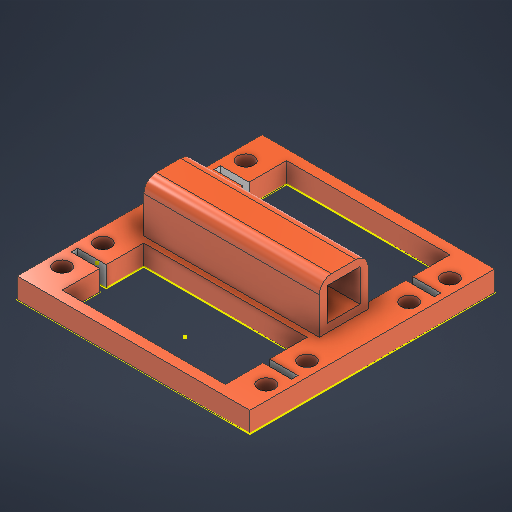
# Autodesk Inventor part: base
Saved by Autodesk Inventor 2027.1 (Build 311270010, 270A)
## iProperties
Created: 2026-08-01
Part Number: base
Material: Ogólny
Document SubType Name: Modeling
Designer: User
Density: 1 g/cm^3
Appearance: Domyślna
Author: User
Autodesk Inventor part; units mm, degrees
ref_plane "YZ Plane" through (0, 0, 0) normal (1, 0, 0) x (0, 1, 0)
ref_plane "XZ Plane" through (0, 0, 0) normal (0, 1, 0) x (-1, 0, 0)
ref_plane "XY Plane" through (0, 0, 0) normal (0, 0, 1) x (1, 0, 0)
sketch "Szkic1" plane through (0, 0, 0) normal (0, 1, 0) x (-1, 0, 0)
  line L0 (0, 0) -> (0, -35)
  circle A0 centre (0, 0) radius 2
  circle A1 centre (0, -35) radius 2
  line L1 (0, 0) -> (0, -35) construction
  line L2 (-25, 0) -> (-25, -35)
  line L3 (25, -35) -> (25, 0)
  arc A2 (25, 0) -> (-25, 0) centre (0, 0) ccw
  arc A3 (-25, -35) -> (25, -35) centre (0, -35) ccw
  line L4 (-20, -45) -> (20, -45)
  line L5 (20, -45) -> (20, -25)
  line L6 (20, -25) -> (-20, -25)
  line L7 (-20, -25) -> (-20, -45)
  line L8 (-20, -45) -> (20, -25) construction
  line L9 (20, -45) -> (-20, -25) construction
  line L10 (0, -17.5) -> (-25, -17.5) construction
  line L11 (0, -35) -> (0, 0)
  circle A4 centre (0, 0) radius 2
  line L12 (0, -35) -> (0, 0) construction
  line L13 (-20, 10) -> (20, 10)
  line L14 (20, 10) -> (20, -10)
  line L15 (20, -10) -> (-20, -10)
  line L16 (-20, 10) -> (20, -10) construction
  line L17 (20, 10) -> (-20, -10) construction
  line L18 (-20, -10) -> (-20, 10)
  line L19 (0, -17.5) -> (-400, -17.5) construction
  line L20 (0, -17.5) -> (400, -17.5) construction
  line L21 (21.5, 12.5) -> (-21.5, 12.5)
  line L22 (-21.5, 12.5) -> (-21.5, -47.5)
  line L23 (-21.5, -47.5) -> (21.5, -47.5)
  line L24 (21.5, -47.5) -> (21.5, 12.5)
  line L25 (21.5, 12.5) -> (-21.5, -47.5) construction
  line L26 (-21.5, 12.5) -> (21.5, -47.5) construction
  line L27 (21.5, -47.5) -> (28.5, -47.5)
  line L28 (28.5, -47.5) -> (28.5, 12.5)
  line L29 (28.5, 12.5) -> (21.5, 12.5)
  line L30 (21.5, 12.5) -> (21.5, -47.5)
  line L31 (20, 10) -> (20, -10)
  line L32 (20, 0) -> (20, -10)
  circle A5 centre (25, -5) radius 2
  line L33 (20, 0) -> (28.5, 0) construction
  circle A6 centre (25, 5) radius 2
  circle A7 centre (-25, -5) radius 2
  circle A8 centre (-25, 5) radius 2
  line L34 (-21.5, -47.5) -> (-21.5, 12.5)
  line L35 (-21.5, -47.5) -> (-28.5, -47.5)
  line L36 (-28.5, -47.5) -> (-28.5, 12.5)
  line L37 (-28.5, 12.5) -> (-21.5, 12.5)
  circle A9 centre (25, -30) radius 2
  circle A10 centre (25, -40) radius 2
  circle A11 centre (-25, -30) radius 2
  circle A12 centre (-25, -40) radius 2
  point P0 (20, -5)
  dimension "d0" = 35
  dimension "d1" = 4
  dimension "d2" = 4
  dimension "d3" = 50
  dimension "d6" = 40
  dimension "d7" = 20
  dimension "d8" = 400
  dimension "d9" = 180
  dimension "d10" = 43
  dimension "d11" = 60
  dimension "d21" = 7
  dimension "d22" = 60
  dimension "d24" = 4
  dimension "d25" = 5
  dimension "d26" = 5
  constraints: 80 end point, 19 symmetric about line, 13 centre point, 8 midpoint, 7 parallel, 5 collinear, 4 coincident, 4 horizontal, 4 perpendicular, 4 point on circle, 4 tangent, 2 vertical, 1 point on line, 8 other
  measures "d0" distance of L0.start L0.end
  measures "d1" diameter of A0
  measures "d2" diameter of A1
  measures "d3" diameter of A3
  measures "d6" distance of L6.end L5.end
  measures "d7" distance of L5.end L4.end
  measures "d8" distance of L10.start L19.end
  measures "d9" angle of L20 L19
  measures "d10" distance of L23.end L22.end
  measures "d11" distance of L22.end L21.end
  measures "d21" distance of L29.end L28.end
  measures "d22" distance of L28.end L27.end
  measures "d24" diameter of A5
  measures "d25" distance from line of L15 A5.centre
  measures "d26" distance of point (20, -5) A5.centre
extrude "Wyciągnięcie proste1" add sketch "Szkic1" against normal blind 5 contours L21 L24 L23 L22
sketch "Szkic2" plane through (-21.5, 0, -47.5) normal (-1, 0, 0) x (0, 0, 1)
  line L0 (22.5, 0) -> (22.5, -5) projected
  line L1 (37.5, 0) -> (37.5, -5) projected
  line L2 (22.5, 0) -> (37.5, 0)
  line L3 (30, 0) -> (30, 6)
  line L4 (36, 12) -> (24, 12)
  line L5 (24, 12) -> (24, 0)
  line L6 (24, 0) -> (36, 0)
  line L7 (36, 0) -> (36, 12)
  line L8 (36, 12) -> (24, 0) construction
  line L9 (24, 12) -> (36, 0) construction
  line L10 (34, 10) -> (26, 10)
  line L11 (26, 10) -> (26, 2)
  line L12 (26, 2) -> (34, 2)
  line L13 (34, 2) -> (34, 10)
  line L14 (34, 10) -> (26, 2) construction
  line L15 (26, 10) -> (34, 2) construction
  point P0 (47.5, 0)
  point P1 (36, 0)
  point P2 (24, 0)
  dimension "d12" = 6
  dimension "d13" = 12
  dimension "d14" = 12
  dimension "d15" = 8
  dimension "d16" = 8
  constraints: 28 end point, 5 midpoint, 4 parallel, 3 horizontal, 2 perpendicular, 1 vertical
  measures "d12" distance of L3.start L3.end
  measures "d13" distance of L6.end L5.end
  measures "d14" distance of L5.end L4.end
  measures "d15" distance of L12.end L11.end
  measures "d16" distance of L11.end L10.end
extrude "Wyciągnięcie proste2" add sketch "Szkic2" against normal up to surface (43 mm away)
fillet "Zaokrąglenie2" radius 3 2 edges at (0, 12, -11.5) (0, 12, -23.5)
extrude "Wyciągnięcie proste3" add sketch "Szkic1" against normal blind 5 contours A2 A8 L37 L22 L35 A3 A12 L2 A11 A7 | L2 A7 A11 A3 A12 L35 L36 L37 A2 A8 | L29 L28 L27 A3 A10 L3 A9 A5 A2 A6 | A2 A6 L3 A5 A9 A3 A10 L27 L24 L29
sketch "Szkic3" plane through (-21.5, 0, -23.5) normal (-1, 0, 0) x (0, 0, 1)
  line L0 (10, 2) -> (2, 2) construction
  line L1 (2, 10) -> (10, 10) construction
  line L2 (10, 2) -> (2, 10) construction
  line L3 (10, 10) -> (10, 2) construction
  line L4 (2, 2) -> (10, 10) construction
  line L5 (2, 10) -> (10, 10) construction
  line L6 (10, 10) -> (10, 2) construction
  line L7 (10, 2) -> (2, 2) construction
  line L8 (2, 2) -> (2, 10) construction
  line L9 (2, 10) -> (10, 2) construction
  line L10 (10, 10) -> (2, 2) construction
  point P0 (23.5, 0)
  point P1 (6, 6)
  constraints: 16 end point, 3 midpoint, 2 parallel, 1 horizontal, 1 perpendicular
sketch "Szkic4" plane through (0, -5, 0) normal (0, -1, 0) x (1, 0, 0)
  line L0 (20, -10) -> (20, 10) projected
  line L1 (20, 0) -> (20, 0.8)
  line L2 (20, 0) -> (22.1856, 0) construction
  line L3 (20, 0.8) -> (27, 0.8)
  line L4 (27, 0.8) -> (27, 0)
  line L5 (20, 10) -> (20, -10)
  line L6 (20, -0.8) -> (27, -0.8)
  line L7 (27, -0.8) -> (27, 0)
  line L8 (20, 10) -> (-20, 10) projected
  line L9 (0, 10) -> (0, -45)
  line L10 (-20, -45) -> (20, -45) projected
  line L11 (28.5, 12.5) -> (28.5, -47.5) projected
  line L12 (28.5, -17.5) -> (-28.5, -17.5)
  line L13 (-28.5, -47.5) -> (-28.5, 12.5) projected
  line L14 (-20, -10) -> (-20, 10)
  line L15 (-20, 0) -> (-20, 0.8)
  line L16 (-20, 0) -> (-22.1856, 0) construction
  line L17 (-20, 0.8) -> (-27, 0.8)
  line L18 (-27, 0.8) -> (-27, 0)
  line L19 (-20, -0.8) -> (-27, -0.8)
  line L20 (-27, -0.8) -> (-27, 0)
  line L21 (20, -25) -> (20, -45)
  line L22 (20, -35) -> (20, -35.8)
  line L23 (20, -35) -> (22.1856, -35) construction
  line L24 (20, -35.8) -> (27, -35.8)
  line L25 (20, -34.2) -> (27, -34.2)
  line L26 (20, -45) -> (20, -25)
  line L27 (20, -45) -> (-20, -45)
  line L28 (-20, -35) -> (-20, -35.8)
  line L29 (-20, -35) -> (-22.1856, -35) construction
  line L30 (-20, -34.2) -> (-27, -34.2)
  line L31 (-20, -25) -> (-20, -45)
  line L32 (-20, -35.8) -> (-27, -35.8)
  line L33 (27, -34.2) -> (27, -35.8)
  line L34 (-27, -34.2) -> (-27, -35.8)
  point P0 (0, 0)
  point P1 (0, -35)
  dimension "d29" = 0.8
  dimension "d30" = 7
  constraints: 60 end point, 33 symmetric about line, 6 point on line, 5 midpoint, 2 horizontal, 2 vertical, 1 perpendicular
  measures "d29" distance of L1.start L1.end
  measures "d30" distance of L1.end L3.end
extrude "Wyciągnięcie proste4" cut sketch "Szkic4" against normal blind 10
sketch "Szkic5" plane through (0, -5, 0) normal (0, -1, 0) x (1, 0, 0)
  line L0 (-20, -35.8) -> (-27, -35.8) projected
  line L1 (-27, -35.8) -> (-27, -34.2) projected
  line L2 (-27, -34.2) -> (-20, -34.2) projected
  line L3 (-20, -34.2) -> (-20, -25) projected
  line L4 (-20, -25) -> (20, -25) projected
  line L5 (20, -25) -> (20, -34.2) projected
  line L6 (20, -34.2) -> (27, -34.2) projected
  line L7 (27, -34.2) -> (27, -35.8) projected
  line L8 (27, -35.8) -> (20, -35.8) projected
  line L9 (20, -35.8) -> (20, -45) projected
  line L10 (20, -45) -> (-20, -45) projected
  line L11 (-20, -45) -> (-20, -35.8) projected
  line L12 (28.5, 12.5) -> (-28.5, 12.5) projected
  line L13 (-28.5, 12.5) -> (-28.5, -47.5) projected
  line L14 (-28.5, -47.5) -> (28.5, -47.5) projected
  line L15 (28.5, -47.5) -> (28.5, 12.5) projected
  circle A0 centre (-25, -40) radius 2 projected
  circle A1 centre (-25, -30) radius 2 projected
  circle A2 centre (-25, -5) radius 2 projected
  circle A3 centre (-25, 5) radius 2 projected
  circle A4 centre (25, 5) radius 2 projected
  circle A5 centre (25, -5) radius 2 projected
  circle A6 centre (25, -30) radius 2 projected
  circle A7 centre (25, -40) radius 2 projected
  line L16 (-27, 0.8) -> (-20, 0.8) projected
  line L17 (-20, 0.8) -> (-20, 10) projected
  line L18 (-20, 10) -> (20, 10) projected
  line L19 (20, 10) -> (20, 0.8) projected
  line L20 (20, 0.8) -> (27, 0.8) projected
  line L21 (27, 0.8) -> (27, -0.8) projected
  line L22 (27, -0.8) -> (20, -0.8) projected
  line L23 (20, -0.8) -> (20, -10) projected
  line L24 (20, -10) -> (-20, -10) projected
  line L25 (-20, -10) -> (-20, -0.8) projected
  line L26 (-20, -0.8) -> (-27, -0.8) projected
  line L27 (-27, -0.8) -> (-27, 0.8) projected
  point P0 (0, 0)
